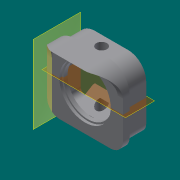
# Autodesk Inventor part: Front
Saved by Autodesk Inventor 2016 (Build 200138000, 138)
## iProperties
Created: 2016-12-22
Part Number: Front
Material: Generic
Document SubType Name: Modeling
Designer: Student
Density: 1 g/cm^3
Appearance: Default
Author: Student
Autodesk Inventor part; units mm, degrees
ref_plane "XZ Plane" through (0, 0, 0) normal (0, 1, 0) x (-1, 0, 0)
ref_plane "XY Plane" through (0, 0, 0) normal (0, 0, 1) x (1, 0, 0)
sketch "Sketch2" plane through (0, 0, 0) normal (0, 0, 1) x (1, 0, 0)
  line L0 (25.1049, -5.6982) -> (25.1049, -19.8714) projected
  arc A0 (22.4633, -22.513) -> (25.1049, -19.8714) centre (22.4633, -19.8714) ccw projected
  line L1 (22.4633, -22.513) -> (2.9815, -22.513) projected
  arc A1 (0.3399, -19.8714) -> (2.9815, -22.513) centre (2.9815, -19.8714) ccw projected
  line L2 (0.3399, -19.8714) -> (0.3399, -5.6982) projected
  arc A2 (6.3851, 0.347) -> (0.3399, -5.6982) centre (6.3851, -5.6982) ccw projected
  line L3 (6.3851, 0.347) -> (19.0597, 0.347) projected
  arc A3 (25.1049, -5.6982) -> (19.0597, 0.347) centre (19.0597, -5.6982) ccw projected
  line L4 (19.0597, 2.506) -> (6.3851, 2.506) projected
  arc A4 (6.3851, 2.506) -> (-1.8191, -5.6982) centre (6.3851, -5.6982) ccw projected
  line L5 (-1.8191, -5.6982) -> (-1.8191, -19.8714) projected
  arc A5 (-1.8191, -19.8714) -> (2.9815, -24.672) centre (2.9815, -19.8714) ccw projected
  line L6 (2.9815, -24.672) -> (22.4633, -24.672) projected
  arc A6 (22.4633, -24.672) -> (27.2639, -19.8714) centre (22.4633, -19.8714) ccw projected
  line L7 (27.2639, -19.8714) -> (27.2639, -5.6982) projected
  arc A7 (27.2639, -5.6982) -> (19.0597, 2.506) centre (19.0597, -5.6982) ccw projected
  line L8 (19.0597, -0.923) -> (6.3851, -0.923)
  arc A8 (6.3851, -0.923) -> (1.6099, -5.6982) centre (6.3851, -5.6982) ccw
  line L9 (1.6099, -5.6982) -> (1.6099, -19.8714)
  arc A9 (1.6099, -19.8714) -> (2.9815, -21.243) centre (2.9815, -19.8714) ccw
  line L10 (2.9815, -21.243) -> (22.4633, -21.243)
  arc A10 (22.4633, -21.243) -> (23.8349, -19.8714) centre (22.4633, -19.8714) ccw
  line L11 (23.8349, -19.8714) -> (23.8349, -5.6982)
  arc A11 (23.8349, -5.6982) -> (19.0597, -0.923) centre (19.0597, -5.6982) ccw
  point P0 (0, 0)
  dimension "d30" = 1.27
  constraints: 8 end point, 8 point on circle, 4 centre point, 7 other
  measures "d30" radial gap between concentric circles of A3 A11
extrude "Extrusion1" add sketch "Sketch2" along normal blind 10.16 contours A7 L7 A6 L6 A5 L5 A4 L4
sketch "Sketch6" plane through (0, 0, 10.16) normal (0, 0, 1) x (1, 0, 0)
  arc A0 (22.4633, -22.513) -> (25.1049, -19.8714) centre (22.4633, -19.8714) ccw projected
  line L0 (22.4633, -22.513) -> (2.9815, -22.513) projected
  arc A1 (0.3399, -19.8714) -> (2.9815, -22.513) centre (2.9815, -19.8714) ccw projected
  line L1 (0.3399, -19.8714) -> (0.3399, -5.6982) projected
  arc A2 (6.3851, 0.347) -> (0.3399, -5.6982) centre (6.3851, -5.6982) ccw projected
  line L2 (6.3851, 0.347) -> (19.0597, 0.347) projected
  arc A3 (25.1049, -5.6982) -> (19.0597, 0.347) centre (19.0597, -5.6982) ccw projected
  line L3 (25.1049, -5.6982) -> (25.1049, -19.8714) projected
  line L4 (19.0597, 2.506) -> (6.3851, 2.506) projected
  arc A4 (6.3851, 2.506) -> (-1.8191, -5.6982) centre (6.3851, -5.6982) ccw projected
  line L5 (-1.8191, -5.6982) -> (-1.8191, -19.8714) projected
  arc A5 (-1.8191, -19.8714) -> (2.9815, -24.672) centre (2.9815, -19.8714) ccw projected
  line L6 (2.9815, -24.672) -> (22.4633, -24.672) projected
  arc A6 (22.4633, -24.672) -> (27.2639, -19.8714) centre (22.4633, -19.8714) ccw projected
  line L7 (27.2639, -19.8714) -> (27.2639, -5.6982) projected
  arc A7 (27.2639, -5.6982) -> (19.0597, 2.506) centre (19.0597, -5.6982) ccw projected
  point P0 (0, 0)
extrude "Extrusion2" add sketch "Sketch6" against normal blind 2.54 contours L0 A1 L1 A2 L2 A3 L3 A0
sketch "Sketch7" plane through (0, 0, 10.16) normal (0, 0, 1) x (1, 0, 0)
  circle A0 centre (12.7224, -11.083) radius 9.2329
  line L0 (27.2639, -19.8714) -> (27.2639, -5.6982) construction
  line L1 (19.0597, 2.506) -> (6.3851, 2.506) construction
  line L2 (2.9815, -24.672) -> (22.4633, -24.672) construction
  line L3 (-1.8191, -5.6982) -> (-1.8191, -19.8714) construction
  line L4 (10.7523, 2.506) -> (10.7523, -24.672) construction
  line L5 (-1.8191, -7.0342) -> (27.2639, -7.0342) construction
  point P0 (0, 0)
  point P1 (12.7224, -7.0342)
  point P2 (10.7523, -11.083)
  dimension "d8" = 18.4658
  constraints: 4 end point, 4 point on line, 2 midpoint, 2 perpendicular, 1 centre point, 1 horizontal alignment, 1 vertical alignment
  measures "d8" diameter of A0
extrude "Extrusion3" cut sketch "Sketch7" against normal up to next
sketch "Sketch8" plane through (0, 0, 10.16) normal (0, 0, 1) x (1, 0, 0)
  circle A0 centre (12.7224, -11.083) radius 9.2329 projected
  circle A1 centre (12.7224, -11.083) radius 9.8425
  point P0 (0, 0)
  dimension "d16" = 19.685
  constraints: 1 centre point, 1 coincident
  measures "d16" diameter of A1
extrude "Extrusion4" cut sketch "Sketch8" against normal blind 1.016
sketch "Sketch9" plane through (0, 0, 10.16) normal (0, 0, 1) x (1, 0, 0)
  line L0 (11.3254, 0.1311) -> (14.1194, 0.1311)
  line L1 (14.1194, 0.1311) -> (14.1194, -3.581)
  line L2 (14.1194, -3.581) -> (11.3254, -3.581)
  line L3 (11.3254, -3.581) -> (11.3254, 0.1311)
  circle A0 centre (12.7224, -11.083) radius 9.8425 projected
  line L4 (15.693, -1.2405) -> (10.0356, -1.2405) construction
  point P0 (0, 0)
  point P1 (12.7224, 0.1311)
  dimension "d19" = 2.794
  dimension "d21" = 1.3716
  constraints: 10 end point, 2 parallel, 2 perpendicular, 1 horizontal, 1 midpoint, 1 tangent, 1 vertical alignment
  measures "d19" distance of L0.start L0.end
  measures "d21" distance between parallel lines of L4 L0
extrude "Extrusion5" cut sketch "Sketch9" against normal blind 3.175 contours L0 L1 A0 L3 | A0 L1 L2 L3 picked at (12.5667, -2.8045)
sketch "Sketch10" plane through (6.3851, 0.347, 0) normal (0, -1, 0) x (1, 0, 0)
  line L0 (12.6746, 7.62) -> (0, 7.62) projected
  line L1 (0, 0) -> (0, 7.62) projected
  line L2 (12.6746, 0) -> (0, 0) projected
  line L3 (12.6746, 0) -> (12.6746, 7.62) projected
  point P0 (-6.3851, 0)
extrude "Extrusion6" add sketch "Sketch10" along normal blind 6.35
sketch "Sketch11" plane through (6.3851, -6.003, 0) normal (-1, 0, 0) x (0, 0, 1)
  line L0 (8.0792, 4.1021) -> (0.254, -0.4699)
  line L1 (7.62, 1.6345) -> (7.62, 4.0466) projected
  line L2 (7.62, 1.6345) -> (7.62, 0) projected
  line L3 (7.62, 0) -> (7.62, 4.064)
  line L4 (7.62, 0) -> (0.762, 0)
  line L5 (0, 0) -> (7.62, 0) projected
  line L6 (7.62, 4.0466) -> (9.144, 4.0466) projected
  line L7 (0.762, 0) -> (7.62, 4.0466)
  point P0 (0, 6.003)
  dimension "d26" = 4.064
  dimension "d27" = 6.858
  constraints: 8 end point, 2 point on line, 3 other
  measures "d26" distance of L2.end L3.end
  measures "d27" distance of L2.end L4.end
extrude "Extrusion7" cut sketch "Sketch11" against normal up to surface (12.6746 mm away) contours L1 L2 L4 L0 | L0 L4 L7 L1
ref_plane "Work Plane2" through (2.9815, -11.083, 0) normal (0, -1, 0) x (1, 0, 0)
mirror "Mirror1" about plane through (2.9815, -11.083, 0) normal (0, -1, 0) of "Extrusion6", "Extrusion7"
sketch "Sketch13" plane through (0, 0, 0) normal (0, 0, -1) x (-1, 0, 0)
  line L0 (-25.1049, -5.6982) -> (-25.1049, -19.8714) projected
  arc A0 (-25.1049, -19.8714) -> (-22.4633, -22.513) centre (-22.4633, -19.8714) ccw projected
  line L1 (-22.4633, -22.513) -> (-2.9815, -22.513) projected
  arc A1 (-2.9815, -22.513) -> (-0.3399, -19.8714) centre (-2.9815, -19.8714) ccw projected
  line L2 (-0.3399, -19.8714) -> (-0.3399, -5.6982) projected
  arc A2 (-0.3399, -5.6982) -> (-6.3851, 0.347) centre (-6.3851, -5.6982) ccw projected
  line L3 (-6.3851, 0.347) -> (-19.0597, 0.347) projected
  arc A3 (-19.0597, 0.347) -> (-25.1049, -5.6982) centre (-19.0597, -5.6982) ccw projected
  line L4 (-19.0597, 2.506) -> (-6.3851, 2.506) projected
  arc A4 (1.8191, -5.6982) -> (-6.3851, 2.506) centre (-6.3851, -5.6982) ccw projected
  line L5 (1.8191, -5.6982) -> (1.8191, -19.8714) projected
  arc A5 (-2.9815, -24.672) -> (1.8191, -19.8714) centre (-2.9815, -19.8714) ccw projected
  line L6 (-2.9815, -24.672) -> (-22.4633, -24.672) projected
  arc A6 (-27.2639, -19.8714) -> (-22.4633, -24.672) centre (-22.4633, -19.8714) ccw projected
  line L7 (-27.2639, -19.8714) -> (-27.2639, -5.6982) projected
  arc A7 (-19.0597, 2.506) -> (-27.2639, -5.6982) centre (-19.0597, -5.6982) ccw projected
  line L8 (-19.0597, -0.161) -> (-6.3851, -0.161)
  arc A8 (-0.8479, -5.6982) -> (-6.3851, -0.161) centre (-6.3851, -5.6982) ccw
  line L9 (-0.8479, -5.6982) -> (-0.8479, -19.8714)
  arc A9 (-2.9815, -22.005) -> (-0.8479, -19.8714) centre (-2.9815, -19.8714) ccw
  line L10 (-2.9815, -22.005) -> (-22.4633, -22.005)
  arc A10 (-24.5969, -19.8714) -> (-22.4633, -22.005) centre (-22.4633, -19.8714) ccw
  line L11 (-24.5969, -19.8714) -> (-24.5969, -5.6982)
  arc A11 (-19.0597, -0.161) -> (-24.5969, -5.6982) centre (-19.0597, -5.6982) ccw
  point P0 (0, 0)
  dimension "d32" = 0.508
  constraints: 8 end point, 8 point on circle, 4 centre point, 7 other
  measures "d32" distance between parallel lines of L3 L8
extrude "Extrusion8" add sketch "Sketch13" against normal up to surface (7.62 mm away) contours A3 L3 A2 L2 A1 L1 A0 L0
sketch "Sketch14" plane through (0, 0, 10.16) normal (0, 0, 1) x (1, 0, 0)
  line L0 (19.0597, 2.506) -> (6.3851, 2.506) projected
  arc A0 (6.3851, 2.506) -> (-1.8191, -5.6982) centre (6.3851, -5.6982) ccw projected
  line L1 (-1.8191, -5.6982) -> (-1.8191, -19.8714) projected
  arc A1 (-1.8191, -19.8714) -> (2.9815, -24.672) centre (2.9815, -19.8714) ccw projected
  line L2 (2.9815, -24.672) -> (22.4633, -24.672) projected
  arc A2 (22.4633, -24.672) -> (27.2639, -19.8714) centre (22.4633, -19.8714) ccw projected
  line L3 (27.2639, -19.8714) -> (27.2639, -5.6982) projected
  arc A3 (27.2639, -5.6982) -> (19.0597, 2.506) centre (19.0597, -5.6982) ccw projected
  line L4 (11.3254, -1.3402) -> (11.3254, 0.1311) projected
  line L5 (11.3254, 0.1311) -> (14.1194, 0.1311) projected
  line L6 (14.1194, 0.1311) -> (14.1194, -1.3402) projected
  arc A4 (11.3254, -1.3402) -> (14.1194, -1.3402) centre (12.7224, -11.083) ccw projected
  line L7 (6.3851, 0.474) -> (19.0597, 0.474)
  arc A5 (25.2319, -5.6982) -> (19.0597, 0.474) centre (19.0597, -5.6982) ccw
  line L8 (25.2319, -5.6982) -> (25.2319, -19.8714)
  arc A6 (22.4633, -22.64) -> (25.2319, -19.8714) centre (22.4633, -19.8714) ccw
  line L9 (22.4633, -22.64) -> (2.9815, -22.64)
  arc A7 (0.2129, -19.8714) -> (2.9815, -22.64) centre (2.9815, -19.8714) ccw
  line L10 (0.2129, -19.8714) -> (0.2129, -5.6982)
  arc A8 (6.3851, 0.474) -> (0.2129, -5.6982) centre (6.3851, -5.6982) ccw
  arc A9 (27.2639, -5.6982) -> (19.0597, 2.506) centre (19.0597, -5.6982) ccw projected
  line L11 (27.2639, -19.8714) -> (27.2639, -5.6982) projected
  line L12 (27.2639, -5.6982) -> (25.2319, -5.6982)
  line L13 (0.2129, -5.6982) -> (-1.8191, -5.6982)
  point P0 (0, 0)
  dimension "d35" = 2.032
  constraints: 12 end point, 8 point on circle, 4 centre point, 2 perpendicular, 7 other
  measures "d35" distance between parallel lines of L0 L7
extrude "Extrusion9" add sketch "Sketch14" along normal blind 6.35 contours A3 L12 A5 L7 A8 L13 A0 L0
sketch "Sketch15" plane through (27.2639, -19.8714, 0) normal (1, 0, 0) x (0, 0, -1)
  line L0 (-10.16, 14.1732) -> (-16.51, 14.1732) projected
  line L1 (-16.51, 22.3774) -> (-16.51, 14.1732) projected
  arc A0 (-10.16, 14.1732) -> (-16.51, 22.3774) centre (-19.3004, 13.6582) ccw
  line L2 (-10.16, 14.1732) -> (-16.51, 14.1732) projected
  point P0 (0, 19.8714)
  constraints: 2 point on circle, 1 centre point
extrude "Extrusion10" cut sketch "Sketch15" against normal through all
sketch "Sketch16" plane through (0, 0, 0) normal (0, 0, -1) x (-1, 0, 0)
  line L0 (-25.1049, -5.6982) -> (-25.1049, -19.8714) projected
  arc A0 (-25.1049, -19.8714) -> (-22.4633, -22.513) centre (-22.4633, -19.8714) ccw projected
  line L1 (-22.4633, -22.513) -> (-2.9815, -22.513) projected
  arc A1 (-2.9815, -22.513) -> (-0.3399, -19.8714) centre (-2.9815, -19.8714) ccw projected
  line L2 (-0.3399, -19.8714) -> (-0.3399, -5.6982) projected
  arc A2 (-0.3399, -5.6982) -> (-6.3851, 0.347) centre (-6.3851, -5.6982) ccw projected
  line L3 (-6.3851, 0.347) -> (-19.0597, 0.347) projected
  arc A3 (-19.0597, 0.347) -> (-25.1049, -5.6982) centre (-19.0597, -5.6982) ccw projected
  line L4 (-19.0597, 2.506) -> (-6.3851, 2.506) projected
  arc A4 (1.8191, -5.6982) -> (-6.3851, 2.506) centre (-6.3851, -5.6982) ccw projected
  line L5 (1.8191, -5.6982) -> (1.8191, -19.8714) projected
  arc A5 (-2.9815, -24.672) -> (1.8191, -19.8714) centre (-2.9815, -19.8714) ccw projected
  line L6 (-2.9815, -24.672) -> (-22.4633, -24.672) projected
  arc A6 (-27.2639, -19.8714) -> (-22.4633, -24.672) centre (-22.4633, -19.8714) ccw projected
  line L7 (-27.2639, -19.8714) -> (-27.2639, -5.6982) projected
  arc A7 (-19.0597, 2.506) -> (-27.2639, -5.6982) centre (-19.0597, -5.6982) ccw projected
  line L8 (-25.9939, -5.6982) -> (-25.9939, -19.8714)
  arc A8 (-25.9939, -19.8714) -> (-22.4633, -23.402) centre (-22.4633, -19.8714) ccw
  line L9 (-22.4633, -23.402) -> (-2.9815, -23.402)
  arc A9 (-2.9815, -23.402) -> (0.5491, -19.8714) centre (-2.9815, -19.8714) ccw
  line L10 (0.5491, -19.8714) -> (0.5491, -5.6982)
  arc A10 (0.5491, -5.6982) -> (-6.3851, 1.236) centre (-6.3851, -5.6982) ccw
  line L11 (-6.3851, 1.236) -> (-19.0597, 1.236)
  arc A11 (-19.0597, 1.236) -> (-25.9939, -5.6982) centre (-19.0597, -5.6982) ccw
  point P0 (0, 0)
  dimension "d40" = 1.27
  constraints: 8 end point, 8 point on circle, 4 centre point, 7 other
  measures "d40" radial gap between concentric circles of A7 A11
extrude "Extrusion11" cut sketch "Sketch16" against normal blind 7.62 contours L4 A4 L5 A5 L6 A6 L7 A7
sketch "Sketch17" plane through (6.3851, 1.236, 0) normal (0, 1, 0) x (1, 0, 0)
  circle A0 centre (6.3373, -3.81) radius 2.032
  line L0 (12.6746, -7.62) -> (0, -7.62) projected
  line L1 (0, 0) -> (0, -7.62) projected
  point P0 (-6.3851, 0)
  point P1 (6.3373, -7.62)
  point P2 (0, -3.81)
  dimension "d43" = 4.064
  dimension "d44" = 3.81
  constraints: 2 midpoint, 1 centre point, 1 horizontal alignment, 1 vertical alignment
  measures "d43" diameter of A0
  measures "d44" distance from line of A0.centre L0
extrude "Extrusion12" cut sketch "Sketch17" against normal blind 6.096
mirror "Mirror2" about plane through (2.9815, -11.083, 0) normal (0, -1, 0) of "Extrusion12"
body "Solid1"
